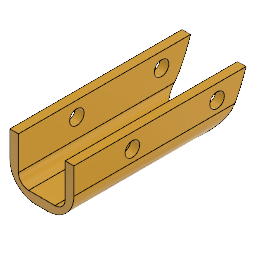
Leg (Autodesk Fusion 360 design; units mm, degrees)
Autodesk Fusion 360 part; units mm, degrees
sketch "Sketch1" plane through (0, 0, 0) normal (0, 0, 1) x (1, 0, 0)
  line L0 (8, -24.5) -> (-8, -24.5)
  line L1 (-8, -24.5) -> (-8, 24.5)
  line L2 (-8, 24.5) -> (8, 24.5)
  line L3 (8, 24.5) -> (8, -24.5)
  line L4 (8, -24.5) -> (-8, 24.5) construction
  line L5 (-8, -24.5) -> (8, 24.5) construction
  line L6 (8, 24.5) -> (11, 24.5)
  line L7 (11, 24.5) -> (11, -24.5)
  line L8 (11, -24.5) -> (8, -24.5)
  line L9 (8, -24.5) -> (8, 24.5)
  line L10 (-8, 24.5) -> (-11, 24.5)
  line L11 (-11, 24.5) -> (-11, -24.5)
  line L12 (-11, -24.5) -> (-8, -24.5)
  line L13 (-8, -24.5) -> (-8, 24.5)
  dimension "d1" = 16
  dimension "d2" = 3
  dimension "d3" = 3
  dimension "d14" = 49
  constraint perpendicular L0 L1
  constraint parallel L0 L2
  constraint parallel L1 L3
  constraint horizontal L0
  constraint coincident L4 origin
  constraint coincident L5 origin
  constraint horizontal L6
  constraint vertical L7
  constraint horizontal L8
  constraint vertical L9
  constraint coincident L0.start L3.end
  constraint horizontal L10
  constraint vertical L11
  constraint horizontal L12
  constraint vertical L13
  constraint coincident L0.end L1.start
  measures "d1" distance of L1.end L2.end
  measures "d2" distance of L2.end L6.end
  measures "d3" distance of L1.end L10.end
  measures "d14" distance of L6.end L7.end
  measures "d24" distance of L0.end
  measures "d25" distance of L0.end
extrude "Extrude2" add sketch "Sketch1" along normal blind 15 contours L3 L6 L7 L8 L9 | L1 L10 L11 L12 L13 makes body 1 at (-11, 8.1667, 5) makes body 2 at (8, 8.1667, 5)
extrude "Extrude1" add sketch "Sketch1" against normal blind 3 bodies 1 2
sketch "Sketch2" plane through (11, 0, 0) normal (1, 0, 0) x (0, 1, 0)
  line L0 (24.5, -3) -> (24.5, 15)
  line L1 (24.5, 15) -> (-24.5, 15)
  line L2 (-24.5, 15) -> (-24.5, -3)
  circle A0 centre (14.5, 10) radius 2.5
  circle A1 centre (-14.5, 10) radius 2.5
  line L3 (-24.5, -3) -> (24.5, -3)
  dimension "d8" = 5
  dimension "d9" = 5
  dimension "d10" = 29
  dimension "d11" = 5
  dimension "d12" = 10
  dimension "d15" = 10
  dimension "d16" = 5
  measures "d8" diameter of A0
  measures "d9" diameter of A1
  measures "d10" horizontal distance of A0.centre A1.centre
  measures "d11" distance of L1 A0.centre
  measures "d12" distance of L0 A0.centre
  measures "d15" horizontal distance of L1.end A1.centre
  measures "d16" vertical distance of L1.end A1.centre
extrude "Extrude3" cut sketch "Sketch2" against normal through all contours A0 | A1 bodies 1
sketch "Sketch3" plane through (0, 0, 0) normal (0, 0, 1) x (1, 0, 0)
  line L0 (4, -30) -> (-4, -30)
  line L1 (-4, -30) -> (-4, 30)
  line L2 (-4, 30) -> (4, 30)
  line L3 (4, 30) -> (4, -30)
  line L4 (4, -30) -> (-4, 30) construction
  line L5 (-4, -30) -> (4, 30) construction
  dimension "d17" = 60
  dimension "d18" = 8
  constraint perpendicular L0 L1
  constraint parallel L0 L2
  constraint parallel L1 L3
  constraint horizontal L0
  constraint coincident L4 origin
  constraint coincident L5 origin
  measures "d17" distance of L0.end L1.end
  measures "d18" distance of L1.end L2.end
extrude "Extrude4" add sketch "Sketch3" along normal blind 8 separate body makes body 3
move_body "Move1" bodies 3 to x (1, 0, 0) y (0, 1, 0) z (0, 0, 1) at (-45, 0, 0)
sketch "Sketch4" plane through (-41, 0, 0) normal (1, 0, 0) x (0, 1, 0)
  line L0 (-30, 0) -> (30, 0)
  line L1 (30, 0) -> (30, 8)
  line L2 (30, 8) -> (-30, 8)
  line L3 (-30, 8) -> (-30, 0)
  circle A0 centre (-9, 4) radius 2.5
  circle A1 centre (20, 4) radius 2.5
  line L4 (-9, 4) -> (20, 4) construction
  dimension "d21" = 5
  dimension "d22" = 5
  dimension "d23" = 29
  dimension "d24" = 10
  dimension "d25" = 4
  constraint coincident A0.centre L4.start
  constraint coincident A1.centre L4.end
  constraint parallel L2 L4
  measures "d21" diameter of A0
  measures "d22" diameter of A1
  measures "d23" horizontal distance of A0.centre A1.centre
  measures "d24" distance of L1 A1.centre
  measures "d25" vertical distance of L1.end A1.centre
extrude "Extrude5" cut sketch "Sketch4" against normal through all contours A0 | A1 bodies 3
extrude "Extrude6" add 1 faces at (-2.6667, -24.5, -2) along direction (0, -1, 0) blind 10 on bodies 1 bodies 1
sketch "Sketch6" plane through (11, 0, 0) normal (1, 0, 0) x (0, 1, 0)
  circle A0 centre (14.5, 10) radius 2.5
  circle A1 centre (-14.5, 10) radius 2.5
  line L0 (-34.5, -3) -> (24.5, -3)
  line L1 (24.5, -3) -> (24.5, 15)
  line L2 (24.5, 15) -> (-34.5, 15)
  line L3 (-34.5, 15) -> (-34.5, -3)
  spline S0 degree 2 poles (5.6166, -3) (19.3532, 0.6042) (24.5, 15) knots 0 0 0 2.762568 2.762568 2.762568 weights 1 1.952038 1
  constraint coincident L1.end L2.start
  constraint coincident L0 S0.start
fillet "Fillet1" radius 3.5 2 edges at (-8, -5, 0) (8, -5, 0) on bodies 1
fillet "Fillet2" radius 9 2 edges at (-11, -5, -3) (11, -5, -3) on bodies 1
extrude "Extrude7" cut sketch "Sketch6" against normal through all contours L0 L1 S0 bodies 1
hidden bodies 3
named bodies: "Body1", "Body2"
